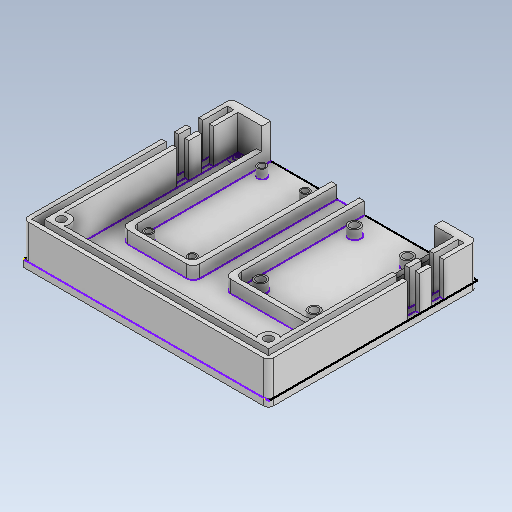
# Autodesk Inventor part: Part1
Saved by Autodesk Inventor 2020.2 (Build 242310000, 310)
## iProperties
Created: 2019-12-02
Part Number: Part1
Material: Generic
Document SubType Name: Modeling
Designer: athiy
Density: 1 g/cm^3
Appearance: Default
Author: athiy
Autodesk Inventor part; units mm, degrees
ref_plane "YZ Plane" through (0, 0, 0) normal (1, 0, 0) x (0, 1, 0)
ref_plane "XZ Plane" through (0, 0, 0) normal (0, 1, 0) x (-1, 0, 0)
ref_plane "XY Plane" through (0, 0, 0) normal (0, 0, 1) x (1, 0, 0)
sketch "Sketch1" plane through (0, 0, 0) normal (0, 1, 0) x (-1, 0, 0)
  line L0 (0, 0) -> (100, 0)
  line L1 (100, 0) -> (100, -85)
  line L2 (100, -85) -> (0, -85)
  line L3 (0, -85) -> (0, 0)
  line L4 (100, -85) -> (100, -81.5)
  line L5 (100, -85) -> (0, -85)
  line L6 (0, 0) -> (100, 0)
  dimension "d0" = 100
  dimension "d1" = 85
  constraints: 14 end point, 4 equal length, 1 horizontal, 1 perpendicular, 1 point on line
  measures "d0" distance of L1.end L2.end
  measures "d1" distance of L0.end L1.end
extrude "Extrusion1" add sketch "Sketch1" along normal blind 3
sketch "Sketch5" plane through (0, 3, 0) normal (0, 1, 0) x (1, 0, 0)
  line L0 (-100, 85.0019) -> (0, 85.0019)
  line L1 (0, 85.0019) -> (0, 0.0019)
  line L2 (0, 0.0019) -> (-100, 0.0019)
  circle A0 centre (-19.0927, 37.6844) radius 1.75
  circle A1 centre (-40.8547, 37.6844) radius 1.75
  circle A2 centre (-19.0927, 75.8444) radius 1.75
  circle A3 centre (-40.8547, 75.8444) radius 1.75
  circle A4 centre (-19.0927, 37.6844) radius 2.3949
  circle A5 centre (-40.8547, 37.6844) radius 2.3949
  line L3 (-29.9737, 32.0144) -> (-16.9737, 32.0144)
  line L4 (-13.9737, 35.0144) -> (-13.9737, 81.5019)
  line L5 (-45.9737, 85) -> (-45.9737, 35.0144)
  line L6 (-42.9737, 32.0144) -> (-29.9737, 32.0144)
  circle A6 centre (-19.0927, 75.8444) radius 2.3949
  circle A7 centre (-40.8547, 75.8444) radius 2.3949
  line L7 (0, 0.0019) -> (0, 3.5019)
  arc A8 (-16.9737, 32.0144) -> (-13.9737, 35.0144) centre (-16.9737, 35.0144) ccw
  arc A9 (-45.9737, 35.0144) -> (-42.9737, 32.0144) centre (-42.9737, 35.0144) ccw
  line L8 (0, 0.0019) -> (-100, 0.0019)
  line L9 (-100, 85.0019) -> (0, 85.0019)
  line L10 (-100, 85) -> (-100, 0)
  line L11 (-100, 85) -> (-100, 0)
  line L12 (0, 81.5019) -> (-13.9774, 81.5019)
  line L13 (0, 85) -> (-100, 85) projected
  line L14 (-13.9774, 81.5019) -> (-13.9774, 85)
  line L15 (0, 0) -> (0, 85) projected
  line L16 (0, 81.5019) -> (0, 85)
  line L17 (0, 85) -> (-13.9774, 85)
  line L18 (-84.1683, 81.5019) -> (-84.1683, 30.8419)
  line L19 (-81.6283, 28.3019) -> (-61.9083, 28.3019)
  line L20 (-59.3683, 30.8419) -> (-59.3683, 85)
  line L21 (-84.1683, 28.3019) -> (-83.1683, 28.3019)
  circle A10 centre (-62.9521, 31.8419) radius 1.27
  circle A11 centre (-80.6721, 31.8419) radius 1.27
  circle A12 centre (-62.9521, 77.9619) radius 1.27
  circle A13 centre (-80.6721, 77.9619) radius 1.27
  circle A14 centre (-62.9521, 31.8419) radius 1.77
  circle A15 centre (-80.6721, 31.8419) radius 1.77
  circle A16 centre (-62.9521, 77.9619) radius 1.77
  circle A17 centre (-80.6721, 77.9619) radius 1.77
  line L22 (0, 81.5019) -> (-6, 81.5019)
  line L23 (-10.7809, 6.0019) -> (-89.1583, 6.0019)
  line L24 (-100, 85) -> (-100, 0) projected
  line L25 (-93.9318, 10.7754) -> (-93.9318, 81.5019)
  line L26 (-100, 0) -> (0, 0) projected
  line L27 (-1.7513, 1.7519) -> (-98.2487, 1.7519)
  line L28 (-98.2487, 81.5019) -> (-98.2487, 0.0019)
  line L29 (-1.7513, 0.0019) -> (-1.7513, 81.5019)
  line L30 (-4.1808, 81.5019) -> (-4.1808, 4.2163)
  line L31 (-4.1808, 4.2163) -> (-95.6828, 4.2163)
  line L32 (-95.6828, 4.2163) -> (-95.6828, 81.5019)
  line L33 (-100, 81.5019) -> (-84.1683, 81.5019)
  line L34 (-84.1683, 85) -> (-84.1683, 81.5019)
  line L35 (-98.2487, 81.5019) -> (-100, 81.5019)
  arc A18 (-61.9083, 28.3019) -> (-59.3683, 30.8419) centre (-61.9083, 30.8419) ccw
  arc A19 (-84.1683, 30.8419) -> (-81.6283, 28.3019) centre (-81.6283, 30.8419) ccw
  line L36 (-47.951, 85) -> (-11.9644, 85)
  line L37 (-11.9644, 81.5019) -> (-11.9644, 32.61)
  line L38 (-14.5044, 30.07) -> (-45.411, 30.07)
  line L39 (-47.951, 32.61) -> (-47.951, 85)
  line L40 (-57.2053, 85) -> (-86.408, 85)
  line L41 (-86.3642, 81.5019) -> (-86.3642, 28.9985)
  line L42 (-83.8242, 26.4585) -> (-59.7453, 26.4585)
  line L43 (-57.2053, 28.9985) -> (-57.2053, 85)
  arc A20 (-14.5044, 30.07) -> (-11.9644, 32.61) centre (-14.5044, 32.61) ccw
  arc A21 (-47.951, 32.61) -> (-45.411, 30.07) centre (-45.411, 32.61) ccw
  arc A22 (-59.7453, 26.4585) -> (-57.2053, 28.9985) centre (-59.7453, 28.9985) ccw
  arc A23 (-86.3642, 28.9985) -> (-83.8242, 26.4585) centre (-83.8242, 28.9985) ccw
  circle A24 centre (-7.75, 7.7519) radius 1.75
  circle A25 centre (-92.1818, 7.7519) radius 1.75
  circle A26 centre (-7.7244, 79.7775) radius 1.7244
  circle A27 centre (-92.1716, 79.7418) radius 1.7602
  line L44 (-6, 81.5019) -> (-6, 10.7828)
  line L45 (-6, 6.035) -> (-6, 6.0019)
  arc A28 (-6, 10.7828) -> (-10.7809, 6.0019) centre (-7.75, 7.7519) ccw
  arc A29 (-89.1583, 6.0019) -> (-93.9318, 10.7754) centre (-92.1818, 7.7519) ccw
  circle A30 centre (-7.7244, 79.7775) radius 3.5026
  circle A31 centre (-92.1716, 79.7418) radius 3.4825
  line L46 (-1.7513, 81.5019) -> (-1.7513, 71.5019)
  line L47 (-1.7513, 71.5019) -> (0, 71.5019)
  line L48 (-4.1808, 61.5019) -> (-6, 61.5019)
  line L49 (0, 71.5019) -> (0, 66.5019)
  line L50 (0, 66.5019) -> (-1.7513, 66.5019)
  line L51 (-1.7513, 66.5019) -> (-1.7513, 61.5019)
  line L52 (-1.7513, 61.5019) -> (0, 61.5019)
  line L53 (-4.1808, 71.5019) -> (-6, 71.5019)
  line L54 (-4.1808, 66.5019) -> (-6, 66.5019)
  line L55 (0, 61.5019) -> (0, 56.5019)
  line L56 (0, 56.5019) -> (-1.7513, 56.5019)
  line L57 (-4.1808, 56.5019) -> (-6, 56.5019)
  line L58 (-98.2487, 56.5019) -> (-100, 56.5019)
  line L59 (-98.2487, 61.5019) -> (-100, 61.5019)
  line L60 (-98.2487, 66.5019) -> (-100, 66.5019)
  line L61 (-98.2487, 71.5019) -> (-100, 71.5019)
  line L62 (-93.9318, 56.5019) -> (-95.6828, 56.5019)
  line L63 (-93.9318, 61.5019) -> (-95.6828, 61.5019)
  line L64 (-93.9318, 66.5019) -> (-95.6828, 66.5019)
  line L65 (-93.9318, 71.5019) -> (-95.6828, 71.5019)
  line L66 (-93.9318, 81.5019) -> (-95.6828, 81.5019)
  point P0 (-13.9737, 32.0144)
  point P1 (-45.9737, 32.0144)
  point P2 (-98.2487, 0.0019)
  point P3 (-93.9318, 76.7368)
  point P4 (-89.1667, 81.5019)
  point P5 (-92.1716, 81.5019)
  point P6 (-95.1766, 81.5019)
  point P7 (-7.7244, 81.5019)
  point P8 (-10.7732, 81.5019)
  point P9 (-6, 76.7287)
  point P10 (0, 71.5019)
  dimension "d22" = 100
  dimension "d23" = 85
  dimension "d30" = 53.2
  dimension "d40" = 6
  dimension "d68" = 10
  dimension "d80" = 24.8
  dimension "d81" = 32
  dimension "d82" = 52.9856
  constraints: 126 end point, 62 point on line, 32 centre point, 27 perpendicular, 25 tangent, 20 point on circle, 12 parallel, 6 coincident, 6 collinear, 5 equal radius, 4 horizontal, 1 vertical
  measures "d22" distance of L1.end L2.end
  measures "d23" distance of L0.end L1.end
  measures "d30" distance of L18.start L21.start
  measures "d40" distance of L12.start L22.end
  measures "d68" distance of L29.end L46.end
  measures "d80" distance of L18.end L20.start
  measures "d81" distance of L5.end L4.start
  measures "d82" distance from line of L13 L6.start
extrude "Extrusion3" add sketch "Sketch5" along normal blind 14 contours L0 L1 L12 A30 L14 | A30 L12
extrude "Extrusion6" add sketch "Sketch5" along normal blind 3.5 contours A4 | A5 | A6 | A7 | A14 | A15 | A16 | A17
extrude "Extrusion7" add sketch "Sketch5" along normal blind 5 contours L0 L43 A22 L42 A23 L41 L33 L18 A19 L19 A18 L20 | L0 L5 A9 L6 L3 A8 L4 L12 L37 A20 L38 A21 L39
extrude "Extrusion10" add sketch "Sketch5" along normal blind 14 contours L0 L34 L33 A31 L10 | L33 L28 L61 L10 | L60 L28 L59 L10 | A31 L33 | L58 L28 L2 L10 | L28 L27 L29 L2 | L29 L56 L1 L2 | L1 L47 L29 L12 | L29 L50 L1 L52
extrude "Extrusion12" add sketch "Sketch5" along normal blind 14 contours L33 A31 L25 L65 L32 | L33 L25 A31 | L64 L25 L63 L32 | L62 L25 A29 L23 A28 L44 L57 L30 L31 L32 | L48 L44 L54 L30 | L30 L53 L44 A30 L12 | A30 L44 L12
fillet "Fillet1" radius 2 4 edges at (-100, 8.5, -85) (-100, 10, -0.0019) (0, 10, -0.0019) (0, 8.5, -85)
fillet "Fillet2" radius 2 1 edges at (0, 1.5, 0)
body "Solid1"
